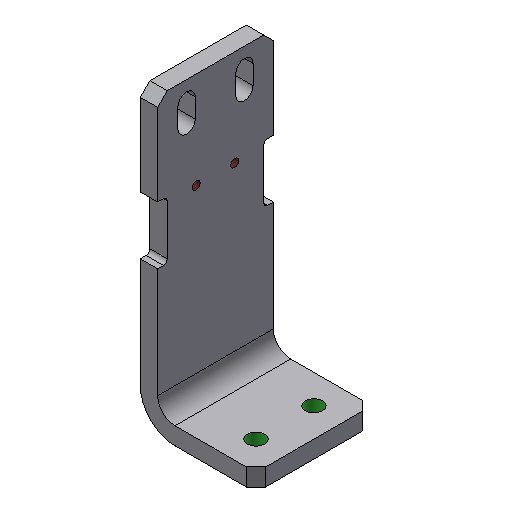
# Autodesk Inventor part: TL20240701-10120CV-022
Saved by Autodesk Inventor 2022.5 (Build 265521000, 521)
## iProperties
Category: FOLLOWER UNIT ASSY
Company: 현대 트랜시스(대유)
Created: 2023-04-11
Part Number: TL20240701-10120CV-022
Checked By: 김형민
Engr Approved By: 김시현
User Status: 2 x18
Material: SS400
Description: 0
Document SubType Name: Modeling
Mfg Approved By: 호상태
Designer: 박성규
Stock Number: 022
Density: 7.85 g/cm^3
Appearance: Painting-RAL7035
Project: SW PJT
DETAIL: Coveryor Assembly
M/C TITLE: CJ 제일제당 협동로봇 포장시스탬 PILOT 장비
PARTS NAME: Bracket
SPECIFICATION: TA20221101-CV200000-015
DocNumber: 221118_Standard_v1
Folder: .\
VDS_Category: 엔지니어링
Detail Description: Processed products
Title: BRACKET
Subject: SW차종 시트조립라인
Author: 박성규
Revision Number: A
Autodesk Inventor part; units mm, degrees
ref_plane "YZ Plane" through (0, 0, 0) normal (1, 0, 0) x (0, 1, 0)
ref_plane "XZ Plane" through (0, 0, 0) normal (0, 1, 0) x (-1, 0, 0)
ref_plane "XY Plane" through (0, 0, 0) normal (0, 0, 1) x (1, 0, 0)
sketch "스케치9" plane through (0, 0, 0) normal (0, 0, 1) x (1, 0, 0)
  line L0 (-30, 76.25) -> (30, 76.25)
  line L1 (30, 76.25) -> (30, -76.25)
  line L2 (30, -76.25) -> (-30, -76.25)
  line L3 (-30, -76.25) -> (-30, 76.25)
  line L4 (-30, 76.25) -> (30, -76.25) construction
  line L5 (30, 76.25) -> (-30, -76.25) construction
  line L6 (-21, 76.25) -> (30, 76.25)
  line L7 (30, 76.25) -> (30, -67.25)
  line L8 (30, -67.25) -> (-21, -67.25)
  line L9 (-21, -67.25) -> (-21, 76.25)
  point P0 (0, 0)
  dimension "d40" = 152.5
  dimension "d41" = 60
  dimension "d42" = 9
  dimension "d43" = 9
  constraints: 20 end point, 4 parallel, 2 horizontal, 2 midpoint, 2 perpendicular, 2 point on line
  measures "d40" distance of L0.end L1.end
  measures "d41" distance of L1.end L2.end
  measures "d42" distance between parallel lines of L3 L9
  measures "d43" distance between parallel lines of L2 L8
extrude "돌출4" add sketch "스케치9" along normal mid plane 60 contours L0 L9 L8 L1 L2 L3
fillet "모깎기2" radius 9 1 edges at (-21, -67.25, 0)
fillet "모깎기3" radius 18 1 edges at (-30, -76.25, 0)
chamfer "모따기1" distance 5 angle 45 4 edges at (-25.5, 76.25, 30) (-25.5, 76.25, -30) (30, -71.75, 30) (30, -71.75, -30)
sketch "스케치10" plane through (-21, -58.25, 30) normal (1, 0, 0) x (0, 0, -1)
  line L0 (55, 134.5) -> (5, 134.5) construction
  line L1 (0, 0) -> (0, 129.5) construction
  line L2 (60, 129.5) -> (60, 0) construction
  line L3 (15, 124.5) -> (15, 114.5) construction
  line L4 (10.5, 124.5) -> (10.5, 114.5)
  line L5 (19.5, 114.5) -> (19.5, 124.5)
  arc A0 (19.5, 124.5) -> (10.5, 124.5) centre (15, 124.5) ccw
  arc A1 (10.5, 114.5) -> (19.5, 114.5) centre (15, 114.5) ccw
  line L6 (45, 124.5) -> (45, 114.5) construction
  line L7 (40.5, 124.5) -> (40.5, 114.5)
  line L8 (49.5, 114.5) -> (49.5, 124.5)
  arc A2 (49.5, 124.5) -> (40.5, 124.5) centre (45, 124.5) ccw
  arc A3 (40.5, 114.5) -> (49.5, 114.5) centre (45, 114.5) ccw
  point P0 (30, 58.25)
  point P1 (15, 119.5)
  point P2 (45, 119.5)
  dimension "d51" = 15
  dimension "d52" = 15
  dimension "d53" = 10
  dimension "d54" = 9
  dimension "d55" = 9
  dimension "d56" = 10
  constraints: 16 end point, 8 point on circle, 8 tangent, 4 centre point, 3 parallel, 2 horizontal alignment, 2 midpoint, 1 vertical
  measures "d51" distance between parallel lines of L2 L6
  measures "d52" distance between parallel lines of L1 L3
  measures "d53" distance from line of L0 L3.start
  measures "d54" distance between parallel lines of L5 L4
  measures "d55" distance between parallel lines of L8 L7
  measures "d56" distance of L6.start L6.end
extrude "돌출5" cut sketch "스케치10" against normal blind 60
sketch "스케치11" plane through (-12, -67.25, 30) normal (0, 1, 0) x (1, 0, 0)
  line L0 (0, 60) -> (37, 60) construction
  line L1 (37, 0) -> (0, 0) construction
  line L2 (42, 55) -> (42, 5) construction
  point P0 (12, 30)
  point P1 (27, 15)
  point P2 (27, 45)
  dimension "d59" = 15
  dimension "d60" = 15
  dimension "d61" = 15
  constraints: 1 vertical alignment
  measures "d59" distance from line of L1 point (27, 15)
  measures "d60" distance from line of L0 point (27, 45)
  measures "d61" distance from line of point (27, 15) L2
hole "구멍3" at (15, -67.25, 15) at (15, -67.25, -15) direction (0, -1, 0) diameter 9 end through all clearance for "Socket Head Cap Screw ISO 4762" size "M8" standard "ISO"
sketch "스케치12" plane through (-30, -58.25, -30) normal (-1, 0, 0) x (0, 0, 1)
  line L0 (5, 134.5) -> (55, 134.5) construction
  point P0 (30, 58.25)
  point P1 (20, 84.5)
  point P2 (40, 84.5)
  dimension "d69" = 10
  dimension "d71" = 50
  dimension "d87" = 20
  dimension "d88" = 10
  constraints: 1 horizontal alignment
  measures "d69" horizontal distance of point (30, 58.25) point (20, 84.5)
  measures "d71" distance from line of L0 point (40, 84.5)
  measures "d87" distance of point (40, 84.5) point (20, 84.5)
  measures "d88" horizontal distance of point (40, 84.5) point (30, 58.25)
hole "구멍4" at (-30, 26.25, -10) at (-30, 26.25, 10) direction (1, 0, 0) diameter 4.134 end through all thread size "M5x0.8" class "6H" standard "TS profile"
sketch "스케치13" plane through (-21, -58.25, 30) normal (1, 0, 0) x (0, 0, -1)
  line L0 (60, 129.5) -> (60, 0) construction
  line L1 (60, 87) -> (55, 87)
  line L2 (55, 87) -> (55, 57)
  line L3 (55, 57) -> (60, 57)
  line L4 (60, 57) -> (60, 87)
  line L5 (0, 129.5) -> (0, 0) construction
  line L6 (0, 87) -> (5, 87)
  line L7 (5, 87) -> (5, 57)
  line L8 (5, 57) -> (0, 57)
  line L9 (0, 57) -> (0, 87)
  line L10 (55, -18) -> (5, -18) construction
  point P0 (30, 58.25)
  point P1 (60, 72)
  dimension "d80" = 5
  dimension "d81" = 5
  dimension "d82" = 30
  dimension "d85" = 90
  constraints: 16 end point, 4 parallel, 4 point on line, 2 horizontal, 2 perpendicular, 1 midpoint
  measures "d80" distance of L1.start L1.end
  measures "d81" distance of L6.start L6.end
  measures "d82" distance of L6.end L7.end
  measures "d85" distance from line of L10 point (60, 72)
extrude "돌출6" cut sketch "스케치13" against normal blind 60
fillet "모깎기4" radius 2 4 edges at (-25.5, -1.25, 25) (-25.5, 28.75, 25) (-25.5, 28.75, -25) (-25.5, -1.25, -25)
equation "\"d43\" = d42"
equation "\"d55\" = d54"
equation "\"d69\" = 0.5 * d87"
equation "\"d81\" = d80"
